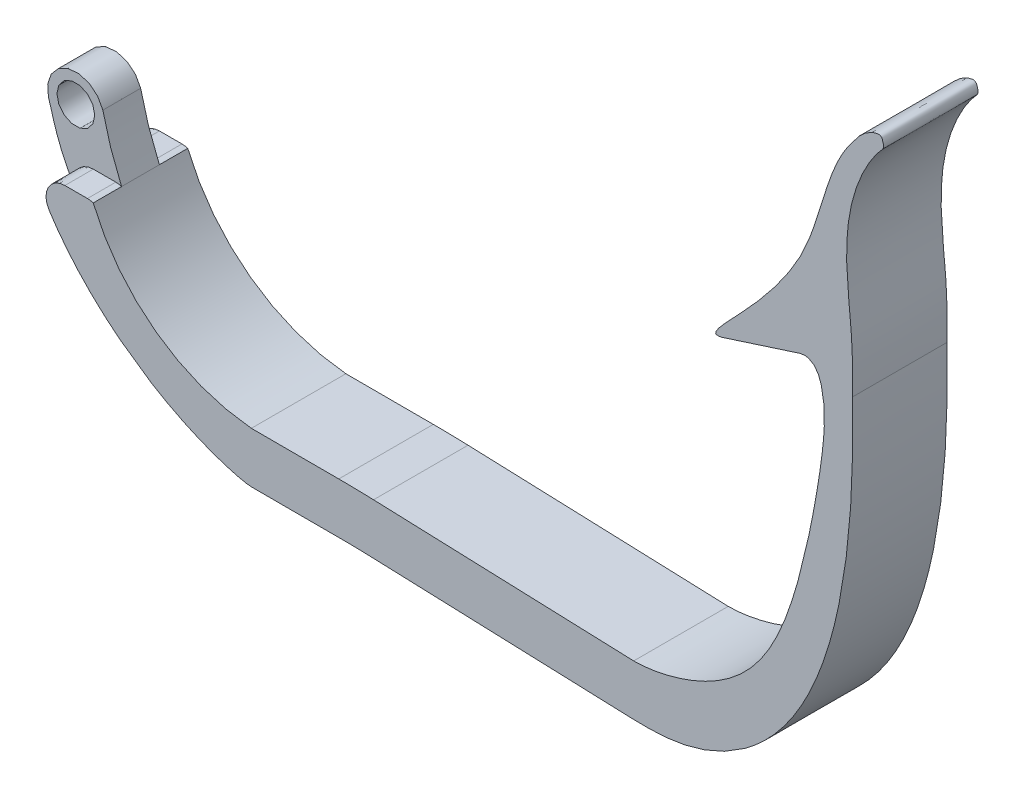
# Autodesk Inventor part: capo2-01
Saved by Autodesk Inventor 2012 (Build 160160000, 160)
## iProperties
Created: 2013-07-31
Part Number: capo2-01
Material: Default
Document SubType Name: Modeling
Designer: Dantro
Density: 1 g/cm^3
Author: Dantro
Autodesk Inventor part; units mm, degrees
note: some values were not read from the file. Chosen so that the rebuilt part matches the saved one: bend side of "Bend Part1".
ref_plane "YZ Plane" through (0, 0, 0) normal (1, 0, 0) x (0, 1, 0)
ref_plane "XZ Plane" through (0, 0, 0) normal (0, 1, 0) x (-1, 0, 0)
ref_plane "XY Plane" through (0, 0, 0) normal (0, 0, 1) x (1, 0, 0)
sketch "Sketch1" plane through (0, 0, 0) normal (0, 0, 1) x (1, 0, 0)
  circle A0 centre (-21.5606, 22.7483) radius 2
  line L0 (48.3905, 39.9137) -> (56.5812, 42.869)
  line L1 (0.0084, 5.3647) -> (40.2906, 5.3016)
  line L2 (0, 0) -> (40.3153, -0.0632)
  circle A1 centre (-21.5606, 22.7483) radius 3
  arc A2 (-16.7192, 17.6514) -> (0.0084, 5.3647) centre (1.7077, 25.2085) ccw
  spline S0 degree 2 poles (-16.7192, 17.6514) (-18.1122, 20.8557) (-18.7036, 23.6633) knots 0 0 0 1 1 1
  line L3 (-16.4416, 17.0127) -> (-16.9969, 18.2901) construction
  arc A3 (-16.938, 18.1638) -> (-16.4938, 17.142) centre (22.0932, 34.5235) ccw construction
  spline S1 degree 4 poles (48.3905, 39.9137) (46.2198, 39.3086) (51.0841, 43.3395) (55.6969, 49.902) (57.6238, 54.5669) (59.2908, 62.016) (61.0837, 64.8276) (62.2971, 66.6601) (64.0952, 67.6712) (64.6285, 67.2924) (64.6366, 66.3773) (64.5298, 66.2561) knots 0 0 0 0 0 0.333246 0.478557 0.629491 0.728891 0.801456 0.874021 0.918879 1 1 1 1 1
  spline S2 degree 4 poles (64.5298, 66.2561) (63.3856, 64.9846) (59.06, 58.041) (62.1645, 48.8813) (62.1141, 44.8499) (62.1769, 41.8484) knots 0 0 0 0 0 0.506064 1 1 1 1 1
  line L4 (65.5562, 67.3967) -> (63.5033, 65.1154) construction
  arc A4 (65.4305, 67.0559) -> (63.8291, 65.2763) centre (68.5384, 62.6487) ccw construction
  line L5 (65.5591, 67.4243) -> (63.5004, 65.0879) construction
  arc A5 (64.4098, 66.2442) -> (64.5264, 66.3766) centre (64.4634, 66.3145) ccw construction
  line L6 (60.0274, 64.0075) -> (64.3917, 68.6054) construction
  arc A6 (64.1614, 67.6269) -> (60.9926, 64.2886) centre (66.1851, 62.5329) ccw construction
  line L7 (57.7429, 56.0515) -> (60.3154, 64.3536) construction
  arc A7 (60.1987, 63.4659) -> (58.1485, 56.8496) centre (96.9718, 48.4455) ccw construction
  line L8 (62.1129, 44.9048) -> (62.2408, 38.7919) construction
  arc A8 (62.1423, 44.2937) -> (62.2446, 39.4038) centre (242.7737, 45.6267) ccw construction
  spline S3 degree 4 poles (62.1769, 41.8484) (62.8309, 30.2941) (61.9423, 8.5733) (50.9255, 0.2265) (43.2835, -0.0431) (40.3153, -0.0632) knots 0 0 0 0 0 0.569368 1 1 1 1 1
  line L9 (45.5741, -0.0276) -> (35.0565, -0.0987) construction
  arc A9 (36.1101, -0.0209) -> (44.5195, 0.0359) centre (39.4695, 125.0779) ccw construction
  line L10 (61.7975, 48.5499) -> (62.5562, 35.1469) construction
  arc A10 (62.3832, 36.4852) -> (61.7766, 47.2006) centre (-85.884, 33.4668) ccw construction
  spline S4 degree 4 poles (56.5812, 42.869) (58.6097, 43.5092) (59.3631, 39.4785) (59.8389, 37.8773) (56.45, 13.8131) (51.2045, 7.7661) (43.2835, 5.3795) (40.2906, 5.3016) knots 0 0 0 0 0 0.253097 0.415308 0.619866 1 1 1 1 1
  line L11 (43.7549, 5.3918) -> (36.8262, 5.2115) construction
  arc A11 (37.6467, 5.6548) -> (42.9125, 5.7918) centre (40.0713, 13.7317) ccw construction
  line L12 (56.4164, 17.3042) -> (50.9496, 8.6156) construction
  arc A12 (51.1594, 9.8278) -> (55.4145, 16.5905) centre (39.0506, 22.1665) ccw construction
  line L13 (51.0766, 41.1317) -> (62.0858, 44.6063) construction
  arc A13 (59.024, 42.2781) -> (54.9201, 40.9829) centre (57.3131, 40.5499) ccw construction
  line L14 (58.8261, 42.6648) -> (59.6138, 36.7091) construction
  arc A14 (59.2933, 37.3215) -> (58.6758, 41.9901) centre (47.5279, 38.1407) ccw construction
  spline S5 degree 4 poles (0, 0) (-1.0361, 0.0038) (-13.3167, 2.7478) (-23.3384, 14.885) (-23.825, 20.1506) (-24.4657, 21.9997) knots 0 0 0 0 0 0.530625 1 1 1 1 1
  line L15 (-23.606, 19.5185) -> (-25.3255, 24.481) construction
  arc A15 (-24.0295, 19.991) -> (-25.3659, 23.8478) centre (-32.5981, 19.1819) ccw construction
  line L16 (0.7697, -0.0028) -> (-0.7697, 0.0028) construction
  arc A16 (-0.5237, 0.1504) -> (0.5248, 0.1466) centre (0.0037, 0.9996) ccw construction
  line L17 (62.6017, 68.4986) -> (66.0417, 66.1268) construction
  arc A17 (64.4723, 66.8293) -> (63.8164, 67.2816) centre (64.0888, 66.975) ccw construction
  point P0 (47.7599, 40.0305)
  point P1 (51.103, 44.1401)
  point P2 (56.0635, 51.286)
  point P3 (59.0291, 60.2025)
  point P4 (64.3217, 67.3127)
  point P5 (61.4059, 59.1637)
  point P6 (61.7454, 48.4623)
  point P7 (62.2096, 66.3065)
  point P8 (56.3114, 8.1089)
  point P9 (46.8004, 0.7606)
  point P10 (59.2199, 39.687)
  point P11 (53.683, 12.9599)
  point P12 (-10.9113, 4.4466)
  point P13 (-22.8583, 17.3121)
  dimension "d32" = 4
  dimension "d45" = 6
  constraints: 36 end point, 30 midpoint, 19 point on circle, 18 centre point, 1 coincident, 1 parallel, 56 other
  measures "d32" diameter of A0
  measures "d45" diameter of A1
extrude "Extrusion2" add sketch "Sketch1" along normal mid plane 10 contours S1 S2 S3 L2 S5 A1 S0 A2 L1 S4 L0 | A1 S5 S0
sketch "Sketch2" plane through (0, 0, 0) normal (1, 0, 0) x (0, 1, 0)
  line L0 (17.6514, -5) -> (23.6633, -5) projected
  line L1 (25.7483, -5) -> (23.6633, -5) projected
  line L2 (17.7483, 2) -> (25.7483, 2)
  line L3 (2.3356, 0) -> (3.712, 0)
  line L4 (17.7483, 2) -> (17.7483, 5)
  line L5 (25.7483, 5) -> (25.7483, 2)
  line L6 (17.7483, 5) -> (25.7483, 5)
  line L7 (17.7483, -2) -> (25.7483, -2)
  line L8 (17.7483, -2) -> (17.7483, -5)
  line L9 (25.7483, -5) -> (25.7483, -2)
  line L10 (17.7483, -5) -> (25.7483, -5)
  point P0 (0, 0)
  point P1 (21.9997, 5)
  point P2 (21.9997, -5)
  dimension "d145" = 2
  dimension "d151" = 8
  constraints: 18 end point, 3 symmetric about line, 2 collinear, 2 parallel, 1 perpendicular
  measures "d145" distance between parallel lines of L2 L3
  measures "d151" distance between parallel lines of L5 L4
extrude "Extrusion3" cut sketch "Sketch2" against normal through all
fillet "Fillet1" radius 2 4 edges at (-16.7612, 17.7483, -3.4979) (-23.0543, 17.7483, -3.4979) (-16.7612, 17.7483, 3.4979) (-23.0543, 17.7483, 3.4979)
sketch "Sketch3" plane through (0, 0, 0) normal (-0.0015668, -0.9999988, 0) x (0.9999988, -0.0015668, 0)
  line L0 (40.3154, 0) -> (40.3154, 5) projected
  line L1 (9.2491, 18.75) -> (9.2491, -16.5064)
  point P0 (0, 0)
  constraints: 2 end point, 1 parallel
bend part "Bend Part1" radius 100 angle 2 line through (9.249, -0.0145, 18.75) along (0, 0, -1) centre toward (-0.0015668, -0.9999988, 0) moving side (0.9999988, -0.0015668, 0) both sides no
body "Solid2"
